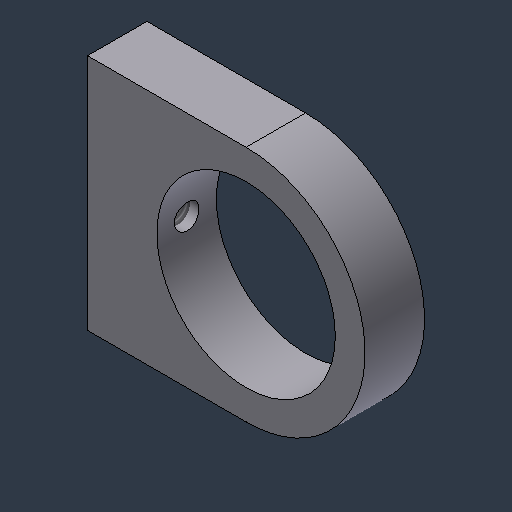
# Autodesk Inventor part: PLATE,BEARING,DRIVE,ELEVATOR
Saved by Autodesk Inventor 2024.3 (Build 283343000, 343)
## iProperties
Category: _
Manager: _
ILogicPurgeVersion: 0.0.0.0
OnSaveVersion: 3.4.3.0
OnSaveAssembly: COREAutomationManager
Created: 2025-01-29
Part Number: PLATE,BEARING,DRIVE,ELEVATOR
Checked By: 00
Engr Approved By: _
User Status: Work In Process
Material: Aluminum, 7075-T6
Description: STANDARD (mm)
Document SubType Name: Modeling
Mfg Approved By: John.Thibert
Designer: John.Thibert
Manufacturer: Standard
Standards Organization: Custom
Density: 2.81 g/cm^3
Appearance: Metal-AL-6061 (Flat)
CN_MASS: 0.0
CN_SERVICEABLE: _
FIRST_DESCRIPTION: _
SECOND_DESCRIPTION: _
THIRD_DESCRIPTION: _
ModelCat: Uncategorized
MaterialName: Aluminum, 7075-T6
Subject: _
Author: John.Thibert
Keywords: -
Revision Number: A
Autodesk Inventor part; units mm, degrees
ref_plane "YZ Plane" through (0, 0, 0) normal (1, 0, 0) x (0, 1, 0)
ref_plane "XZ Plane" through (0, 0, 0) normal (0, 1, 0) x (-1, 0, 0)
ref_plane "XY Plane" through (0, 0, 0) normal (0, 0, 1) x (1, 0, 0)
sketch "Sketch2" plane through (0, 0, 0) normal (0, 0, 1) x (1, 0, 0)
  line L0 (-12.7, 19.05) -> (12.7, 19.05)
  line L1 (12.7, 19.05) -> (12.7, -19.05) construction
  line L2 (12.7, -19.05) -> (-12.7, -19.05)
  line L3 (-12.7, -19.05) -> (-12.7, 19.05)
  line L4 (-12.7, 19.05) -> (12.7, -19.05) construction
  line L5 (12.7, 19.05) -> (-12.7, -19.05) construction
  arc A0 (12.7, -19.05) -> (12.7, 19.05) centre (12.7, 0) ccw
  point P0 (0, 0)
  point P1 (31.75, 0)
  dimension "d0" = 38.1
  dimension "d1" = 25.4
  dimension "d4" = 44.45
  constraints: 12 end point, 3 point on circle, 2 midpoint, 2 parallel, 2 tangent, 1 centre point, 1 horizontal, 1 perpendicular
  measures "d0" distance of L2.end L0.start
  measures "d1" distance of L1.end L2.end
  measures "d4" distance from line of point (31.75, 0) L3
extrude "Extrusion1" add sketch "Sketch2" along normal mid plane 9.525
sketch "Sketch3" plane through (0, 0, -4.7625) normal (0, 0, -1) x (-1, 0, 0)
  arc A0 (-12.7, 19.05) -> (-12.7, -19.05) centre (-12.7, 0) ccw construction
  point P0 (0, 0)
  constraints: 1 coincident
hole "Hole1" at (12.7, 0, -4.7625) direction (0, 0, 1) diameter 28.575 end through all
sketch "Sketch4" plane through (-12.7, -19.05, 4.7625) normal (-1, 0, 0) x (0, 0, 1)
  line L0 (-4.7625, 6.35) -> (-4.7625, 31.75) construction
  point P0 (-4.7625, 19.05)
  point P1 (-4.7625, 19.05)
  dimension "d12" = 25.4
  constraints: 3 coincident, 2 end point, 1 midpoint, 1 vertical
  measures "d12" distance of L0.start L0.end
hole "Hole2" at (-12.7, -12.7, 0) at (-12.7, 12.7, 0) at (-12.7, 0, 0) direction (1, 0, 0) diameter 3.9624 depth 13.6144 tip angle 118 thread size "10-32 UNF" class "2B" standard "ANSI Unified Screw Threads"
body "Solid1"
